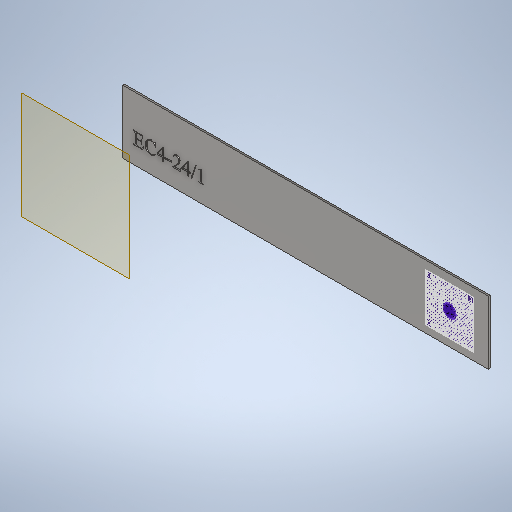
# Autodesk Inventor part: Fechamento
Saved by Autodesk Inventor 2025 (Build 290162000, 162)
## iProperties
Created: 2024-05-06
Part Number: Fechamento
Material: Steel, Alloy
Document SubType Name: Modeling
Designer: 082220005
Density: 7.73 g/cm^3
Appearance: Semi-Polished
Author: 082220005
Autodesk Inventor part; units mm, degrees
note: some values were not read from the file. Chosen so that the rebuilt part matches the saved one: direction of "Emboss2".
ref_plane "YZ Plane" through (0, 0, 0) normal (1, 0, 0) x (0, 1, 0)
ref_plane "XZ Plane" through (0, 0, 0) normal (0, 1, 0) x (-1, 0, 0)
ref_plane "XY Plane" through (0, 0, 0) normal (0, 0, 1) x (1, 0, 0)
sketch "Sketch1" plane through (0, 0, 0) normal (0, 0, 1) x (1, 0, 0)
  line L0 (0, 0) -> (75, 0)
  line L1 (75, 0) -> (75, 13)
  line L2 (75, 13) -> (0, 13)
  line L3 (0, 13) -> (0, 0)
  dimension "d0" = 75
  dimension "d1" = 13
  constraints: 8 end point, 3 perpendicular, 1 horizontal
  measures "d0" distance of L0.start L0.end
  measures "d1" distance of L0.end L1.end
extrude "Extrusion1" add sketch "Sketch1" along normal blind 0.3556
ref_plane "Work Plane4" through (0, 0, 10.1056) normal (0, 0, 1) x (1, 0, 0)
sketch "Sketch4" plane through (0, 0, 10.1056) normal (0, 0, 1) x (1, 0, 0)
  line L0 (2.0314, 6.2186) -> (119.5478, 6.2186) construction
  line L1 (119.5478, 6.2186) -> (119.5478, -15.2193) construction
  line L2 (119.5478, -15.2193) -> (2.0314, -15.2193) construction
  line L3 (2.0314, -15.2193) -> (2.0314, 6.2186) construction
  line L4 (2.8324, 5.9551) -> (2.8324, 4.9528)
  line L5 (2.8324, 4.9528) -> (3.3907, 4.9528)
  spline S0 degree 2 poles (3.3907, 4.9528) (3.6085, 4.9528) (3.6812, 5.0192) knots 0 0 0 1 1 1
  spline S1 degree 2 poles (3.6812, 5.0192) (3.7808, 5.1043) (3.7912, 5.3222) knots 0 0 0 1 1 1
  line L6 (3.7912, 5.3222) -> (3.8596, 5.3222)
  line L7 (3.8596, 5.3222) -> (3.8596, 4.4361)
  line L8 (3.8596, 4.4361) -> (3.7912, 4.4361)
  spline S2 degree 2 poles (3.7912, 4.4361) (3.7642, 4.6208) (3.7393, 4.6726) knots 0 0 0 1 1 1
  spline S3 degree 2 poles (3.7393, 4.6726) (3.704, 4.7391) (3.5504, 4.8138) (3.3907, 4.8138) knots 0 0 0 1 2 2 2
  line L9 (3.3907, 4.8138) -> (2.8324, 4.8138)
  line L10 (2.8324, 4.8138) -> (2.8324, 3.9775)
  spline S4 degree 2 poles (2.8324, 3.9775) (2.8324, 3.8094) (2.8615, 3.7367) (2.9383, 3.6932) (3.042, 3.6932) knots 0 0 0 1 2 3 3 3
  line L11 (3.042, 3.6932) -> (3.4737, 3.6932)
  spline S5 degree 2 poles (3.4737, 3.6932) (3.6895, 3.6932) (3.8845, 3.7533) (3.9738, 3.8405) knots 0 0 0 1 2 2 2
  spline S6 degree 2 poles (3.9738, 3.8405) (4.09, 3.9567) (4.2124, 4.1912) knots 0 0 0 1 1 1
  line L12 (4.2124, 4.1912) -> (4.2871, 4.1912)
  line L13 (4.2871, 4.1912) -> (4.0672, 3.5541)
  line L14 (4.0672, 3.5541) -> (2.1103, 3.5541)
  line L15 (2.1103, 3.5541) -> (2.1103, 3.6226)
  line L16 (2.1103, 3.6226) -> (2.1995, 3.6226)
  spline S7 degree 2 poles (2.1995, 3.6226) (2.2908, 3.6226) (2.3697, 3.6662) knots 0 0 0 1 1 1
  spline S8 degree 2 poles (2.3697, 3.6662) (2.4299, 3.6973) (2.4734, 3.8177) (2.4734, 4.0044) knots 0 0 0 1 2 2 2
  line L17 (2.4734, 4.0044) -> (2.4734, 5.6521)
  spline S9 degree 2 poles (2.4734, 5.6521) (2.4734, 5.8949) (2.4257, 5.9509) knots 0 0 0 1 1 1
  spline S10 degree 2 poles (2.4257, 5.9509) (2.3572, 6.0257) (2.1995, 6.0257) knots 0 0 0 1 1 1
  line L18 (2.1995, 6.0257) -> (2.1103, 6.0257)
  line L19 (2.1103, 6.0257) -> (2.1103, 6.0941)
  line L20 (2.1103, 6.0941) -> (4.0692, 6.0941)
  line L21 (4.0692, 6.0941) -> (4.0962, 5.5359)
  line L22 (4.0962, 5.5359) -> (4.0236, 5.5359)
  spline S11 degree 2 poles (4.0236, 5.5359) (3.9842, 5.7372) (3.8887, 5.8866) (3.7953, 5.926) knots 0 0 0 1 2 2 2
  spline S12 degree 2 poles (3.7953, 5.926) (3.7206, 5.9551) (3.5297, 5.9551) knots 0 0 0 1 1 1
  line L23 (3.5297, 5.9551) -> (2.8324, 5.9551)
  line L24 (6.6839, 6.1522) -> (6.742, 5.289)
  line L25 (6.742, 5.289) -> (6.6839, 5.289)
  spline S13 degree 2 poles (6.6839, 5.289) (6.5677, 5.677) (6.1382, 6.0194) (5.8373, 6.0194) knots 0 0 0 1 2 2 2
  spline S14 degree 2 poles (5.8373, 6.0194) (5.5862, 6.0194) (5.1794, 5.7621) (4.945, 5.1997) (4.945, 4.7806) knots 0 0 0 1 2 3 3 3
  spline S15 degree 2 poles (4.945, 4.7806) (4.945, 4.4361) (5.1649, 3.9297) (5.609, 3.66) (5.8912, 3.66) knots 0 0 0 1 2 3 3 3
  spline S16 degree 2 poles (5.8912, 3.66) (6.1382, 3.66) (6.5159, 3.8716) (6.742, 4.1871) knots 0 0 0 1 2 2 2
  line L26 (6.742, 4.1871) -> (6.8001, 4.1497)
  spline S17 degree 2 poles (6.8001, 4.1497) (6.6092, 3.8115) (6.1008, 3.496) (5.7501, 3.496) knots 0 0 0 1 2 2 2
  spline S18 degree 2 poles (5.7501, 3.496) (5.1193, 3.496) (4.7727, 3.965) knots 0 0 0 1 1 1
  spline S19 degree 2 poles (4.7727, 3.965) (4.5154, 4.3136) (4.5154, 4.7847) knots 0 0 0 1 1 1
  spline S20 degree 2 poles (4.5154, 4.7847) (4.5154, 5.1645) (4.8557, 5.8015) (5.4534, 6.1522) (5.8061, 6.1522) knots 0 0 0 1 2 3 3 3
  spline S21 degree 2 poles (5.8061, 6.1522) (6.0801, 6.1522) (6.3478, 6.0174) knots 0 0 0 1 1 1
  spline S22 degree 2 poles (6.3478, 6.0174) (6.4266, 5.9758) (6.4598, 5.9758) knots 0 0 0 1 1 1
  spline S23 degree 2 poles (6.4598, 5.9758) (6.5117, 5.9758) (6.5491, 6.0111) knots 0 0 0 1 1 1
  spline S24 degree 2 poles (6.5491, 6.0111) (6.5968, 6.063) (6.6175, 6.1522) knots 0 0 0 1 1 1
  line L27 (6.6175, 6.1522) -> (6.6839, 6.1522)
  line L28 (8.7197, 4.49) -> (8.7197, 4.2244)
  line L29 (8.7197, 4.2244) -> (8.3793, 4.2244)
  line L30 (8.3793, 4.2244) -> (8.3793, 3.5541)
  line L31 (8.3793, 3.5541) -> (8.0701, 3.5541)
  line L32 (8.0701, 3.5541) -> (8.0701, 4.2244)
  line L33 (8.0701, 4.2244) -> (6.9931, 4.2244)
  line L34 (6.9931, 4.2244) -> (6.9931, 4.4631)
  line L35 (6.9931, 4.4631) -> (8.1739, 6.146)
  line L36 (8.1739, 6.146) -> (8.3793, 6.146)
  line L37 (8.3793, 6.146) -> (8.3793, 4.49)
  line L38 (8.3793, 4.49) -> (8.7197, 4.49)
  line L39 (8.0701, 4.49) -> (8.0701, 5.7517)
  line L40 (8.0701, 5.7517) -> (7.1778, 4.49)
  line L41 (7.1778, 4.49) -> (8.0701, 4.49)
  line L42 (9.0081, 4.5564) -> (9.9793, 4.5564)
  line L43 (9.9793, 4.5564) -> (9.9793, 4.2742)
  line L44 (9.9793, 4.2742) -> (9.0081, 4.2742)
  line L45 (9.0081, 4.2742) -> (9.0081, 4.5564)
  line L46 (11.8905, 4.0418) -> (11.7121, 3.5541)
  line L47 (11.7121, 3.5541) -> (10.2138, 3.5541)
  line L48 (10.2138, 3.5541) -> (10.2138, 3.6226)
  spline S25 degree 2 poles (10.2138, 3.6226) (10.8758, 4.2265) (11.4153, 4.9901) (11.4153, 5.3076) knots 0 0 0 1 2 2 2
  spline S26 degree 2 poles (11.4153, 5.3076) (11.4153, 5.5484) (11.1186, 5.8596) (10.9131, 5.8596) knots 0 0 0 1 2 2 2
  spline S27 degree 2 poles (10.9131, 5.8596) (10.7243, 5.8596) (10.4275, 5.6397) (10.3549, 5.428) knots 0 0 0 1 2 2 2
  line L49 (10.3549, 5.428) -> (10.2864, 5.428)
  spline S28 degree 2 poles (10.2864, 5.428) (10.3342, 5.7746) (10.7201, 6.146) (11.0107, 6.146) knots 0 0 0 1 2 2 2
  spline S29 degree 2 poles (11.0107, 6.146) (11.3199, 6.146) (11.7349, 5.7497) (11.7349, 5.4799) knots 0 0 0 1 2 2 2
  spline S30 degree 2 poles (11.7349, 5.4799) (11.7349, 5.2869) (11.6457, 5.0939) knots 0 0 0 1 1 1
  spline S31 degree 2 poles (11.6457, 5.0939) (11.5066, 4.7909) (11.1953, 4.4506) knots 0 0 0 1 1 1
  spline S32 degree 2 poles (11.1953, 4.4506) (10.7284, 3.9422) (10.6122, 3.8364) knots 0 0 0 1 1 1
  line L50 (10.6122, 3.8364) -> (11.2763, 3.8364)
  spline S33 degree 2 poles (11.2763, 3.8364) (11.4796, 3.8364) (11.6415, 3.8654) (11.7722, 3.9588) (11.822, 4.0418) knots 0 0 0 1 2 3 3 3
  line L51 (11.822, 4.0418) -> (11.8905, 4.0418)
  line L52 (13.837, 4.49) -> (13.837, 4.2244)
  line L53 (13.837, 4.2244) -> (13.4967, 4.2244)
  line L54 (13.4967, 4.2244) -> (13.4967, 3.5541)
  line L55 (13.4967, 3.5541) -> (13.1875, 3.5541)
  line L56 (13.1875, 3.5541) -> (13.1875, 4.2244)
  line L57 (13.1875, 4.2244) -> (12.1105, 4.2244)
  line L58 (12.1105, 4.2244) -> (12.1105, 4.4631)
  line L59 (12.1105, 4.4631) -> (13.2913, 6.146)
  line L60 (13.2913, 6.146) -> (13.4967, 6.146)
  line L61 (13.4967, 6.146) -> (13.4967, 4.49)
  line L62 (13.4967, 4.49) -> (13.837, 4.49)
  line L63 (13.1875, 4.49) -> (13.1875, 5.7517)
  line L64 (13.1875, 5.7517) -> (12.2952, 4.49)
  line L65 (12.2952, 4.49) -> (13.1875, 4.49)
  line L66 (15.0427, 6.2186) -> (14.1234, 3.5023)
  line L67 (14.1234, 3.5023) -> (13.974, 3.5023)
  line L68 (13.974, 3.5023) -> (14.8933, 6.2186)
  line L69 (14.8933, 6.2186) -> (15.0427, 6.2186)
  line L70 (15.4847, 5.8451) -> (16.1031, 6.146)
  line L71 (16.1031, 6.146) -> (16.1654, 6.146)
  line L72 (16.1654, 6.146) -> (16.1654, 4.0024)
  spline S34 degree 2 poles (16.1654, 4.0024) (16.1654, 3.7886) (16.2006, 3.6828) (16.3127, 3.6268) (16.4849, 3.6226) knots 0 0 0 1 2 3 3 3
  line L73 (16.4849, 3.6226) -> (16.4849, 3.5541)
  line L74 (16.4849, 3.5541) -> (15.5304, 3.5541)
  line L75 (15.5304, 3.5541) -> (15.5304, 3.6226)
  spline S35 degree 2 poles (15.5304, 3.6226) (15.7109, 3.6268) (15.8147, 3.6807) (15.8562, 3.772) (15.8562, 4.0024) knots 0 0 0 1 2 3 3 3
  line L76 (15.8562, 4.0024) -> (15.8562, 5.372)
  spline S36 degree 2 poles (15.8562, 5.372) (15.8562, 5.65) (15.8375, 5.7289) knots 0 0 0 1 1 1
  spline S37 degree 2 poles (15.8375, 5.7289) (15.825, 5.7891) (15.7545, 5.8451) (15.7068, 5.8451) knots 0 0 0 1 2 2 2
  spline S38 degree 2 poles (15.7068, 5.8451) (15.6362, 5.8451) (15.5138, 5.787) knots 0 0 0 1 1 1
  line L77 (15.5138, 5.787) -> (15.4847, 5.8451)
  point P0 (0, 0)
  constraints: 2 other
emboss "Emboss2" sketch "Sketch4" operation cut depth 0.3 direction (0, 0, -1)
sketch "Sketch5" plane through (0, 0, 0.3556) normal (0, 0, 1) x (1, 0, 0)
  line L0 (62.0486, 11.3938) -> (72.0486, 11.3938) construction
  line L1 (72.0486, 11.3938) -> (72.0486, 1.3938) construction
  line L2 (72.0486, 1.3938) -> (62.0486, 1.3938) construction
  line L3 (62.0486, 1.3938) -> (62.0486, 11.3938) construction
  point P0 (0, 0)
  dimension "d36" = 10
  constraints: 2 other
  measures "d36" distance of L0.start L0.end
decal "Decal2"
body "Solid1"
